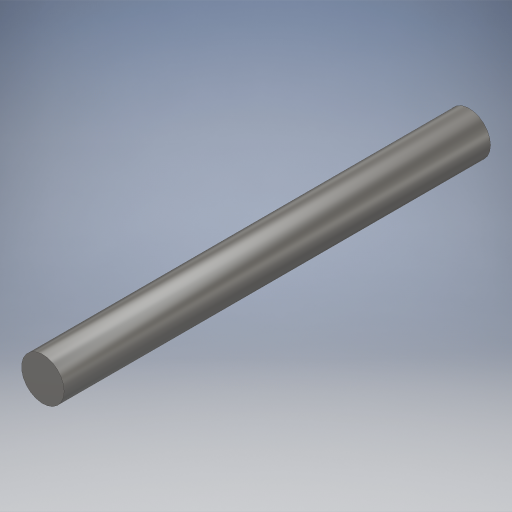
# Autodesk Inventor part: BT805_goteln20_22
Saved by Autodesk Inventor 2023 (Build 270158000, 158)
## iProperties
Company: HTBLA Kaindorf
RuleStatus: InUse
Created: 2023-01-12
Part Number: BT805_goteln20_22
Project: Zeichenmaschine_neu
Material: Edelstahl
Description: getriebe_welle
Document SubType Name: Modeling
Designer: goteln20
Density: 8 g/cm^3
Appearance: Halbpoliert
Mass: 0.502655 g
Surface Area: 1.31947 cm^2
Volume: 0.0628319 cm^3
AfterDocNew0: iProperties-Editor_aufrufen
Author: eligo
Keywords: 22
Autodesk Inventor part; units mm, degrees
ref_plane "YZ Plane" through (0, 0, 0) normal (1, 0, 0) x (0, 1, 0)
ref_plane "XZ Plane" through (0, 0, 0) normal (0, 1, 0) x (-1, 0, 0)
ref_plane "XY Plane" through (0, 0, 0) normal (0, 0, 1) x (1, 0, 0)
sketch "Skizze3" plane through (0, 0, 0) normal (0, 0, 1) x (1, 0, 0)
  line L0 (-16.2553, 0) -> (16.2553, 0)
  line L1 (-10, 0) -> (-10, 1)
  line L2 (-10, 1) -> (10, 1)
  line L3 (10, 1) -> (10, 0)
  point P0 (0, 0)
  point P1 (0, 0)
  point P2 (0, 1)
  dimension "d4" = 2
  dimension "d5" = 20
  constraints: 8 end point, 3 perpendicular, 2 midpoint, 2 point on line, 1 coincident, 1 horizontal, 1 vertical alignment
  measures "d4" diameter of L2 L0
  measures "d5" distance of L1.end L2.end
revolve "Umdrehung1" add sketch "Skizze3" angle 360 about axis through (-16.2553, 0, 0) along (1, 0, 0)
